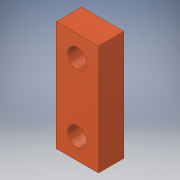
# Autodesk Inventor part: carriage Belt clamp
Saved by Autodesk Inventor 2018 (Build 220112000, 112)
## iProperties
Created: 2013-09-29
Part Number: carriage Belt clamp
Material: ABS Plastic
Document SubType Name: Modeling
Designer: Gabriel Smolnycki
Mass: 1.4513 g
Surface Area: 10.5803 cm^2
Volume: 1.36915 cm^3
Density: 1.06 g/cm^3
Appearance: Smooth - Light Orange
Author: Gabriel Smolnycki
Sending System: SolidWorks 2017
Last Author: Gabriel Smolnycki
Last Saved: 2017-09-14
Autodesk Inventor part; units mm, degrees
ref_plane "YZ Plane" through (0, 0, 0) normal (1, 0, 0) x (0, 1, 0)
ref_plane "XY Plane" through (0, 0, 0) normal (0, 0, 1) x (1, 0, 0)
ref_plane "Work Plane1" through (0, 13, 0) normal (0, 1, 0) x (-1, 0, 0)
sketch "Sketch1" plane through (0, 13, 0) normal (0, 1, 0) x (-1, 0, 0)
  line L0 (5, 6) -> (5, 0)
  line L1 (-5, 6) -> (5, 6)
  line L2 (-5, 0) -> (5, 0)
  line L3 (-5, 6) -> (-5, 0)
  constraints: 8 end point, 2 horizontal, 2 vertical
extrude "Extrusion1" add sketch "Sketch1" against normal blind 26
hole "Hole2" at (0, -8, 0) direction (0, 0, 1) diameter 4.5 depth 6 tip angle 118
sketch "Sketch2" plane through (0, 0, 0) normal (0, 0, 1) x (1, 0, 0)
  point P0 (0, -8)
hole "Hole1" at (0, 8, 0) direction (0, 0, 1) diameter 4.5 depth 6 tip angle 118
sketch "Sketch3" plane through (0, 0, 0) normal (0, 0, 1) x (1, 0, 0)
  point P0 (0, 8)
body "Solid3"
